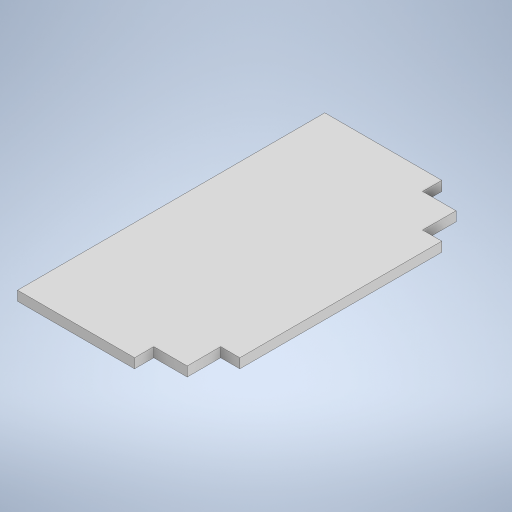
# Autodesk Inventor part: Swerve_cover_1
Saved by Autodesk Inventor 2024 (Build 280153000, 153)
## iProperties
Created: 2023-11-29
Part Number: Swerve_cover_1
Material: Generic
Document SubType Name: Modeling
Designer: s137416
Density: 1 g/cm^3
Appearance: Default
Author: s137416
Autodesk Inventor part; units mm, degrees
ref_plane "YZ Plane" through (0, 0, 0) normal (1, 0, 0) x (0, 1, 0)
ref_plane "XZ Plane" through (0, 0, 0) normal (0, 1, 0) x (-1, 0, 0)
ref_plane "XY Plane" through (0, 0, 0) normal (0, 0, 1) x (1, 0, 0)
sketch "Sketch1" plane through (0, 0, 0) normal (0, 1, 0) x (-1, 0, 0)
  line L0 (140.0646, 47.6727) -> (-14.745, 47.6727)
  line L1 (-84.341, -21.9233) -> (-84.341, -289.1313)
  line L2 (-14.745, -358.7273) -> (140.0646, -358.7273)
  line L3 (140.0646, -358.7273) -> (140.0646, 47.6727)
  line L4 (-14.745, 47.6727) -> (-14.745, 22.2727)
  line L5 (-84.341, -21.9233) -> (-58.941, -21.9233)
  line L6 (-14.745, 22.2727) -> (-58.941, 22.2727)
  line L7 (-58.941, 22.2727) -> (-58.941, -21.9233)
  line L8 (-58.941, -333.3273) -> (-14.745, -333.3273)
  line L9 (-14.745, -333.3273) -> (-14.745, -358.7273)
  line L10 (-58.941, -333.3273) -> (-58.941, -289.1313)
  line L11 (-58.941, -289.1313) -> (-84.341, -289.1313)
  point P0 (0, 0)
  dimension "d1" = 406.4
  dimension "d2" = 25.4
  dimension "d3" = 69.596
  dimension "d4" = 25.4
  dimension "d6" = 69.596
  constraints: 24 end point, 4 perpendicular, 2 horizontal, 2 parallel
  measures "d1" distance between parallel lines of L2 L0
  measures "d2" distance of L0.end L4.end
  measures "d3" distance between parallel lines of L1 L4
  measures "d4" distance of L1.start L5.end
  measures "d6" distance between parallel lines of L0 L5
extrude "Extrusion1" add sketch "Sketch1" along normal blind 12.7
body "Solid1"
